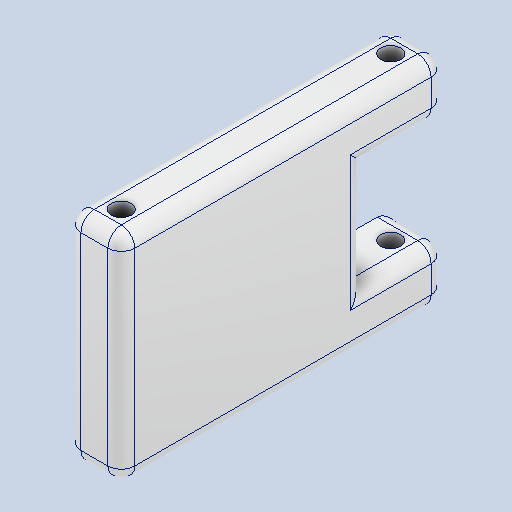
# Autodesk Inventor part: swing pusher
Saved by Autodesk Inventor 2023 (Build 270158000, 158)
## iProperties
Created: 2023-01-25
Part Number: swing pusher
Material: Aluminum 6061
Document SubType Name: Modeling
Designer: Gabriel - T3 CAD
Density: 2.7 g/cm^3
Appearance: Aluminum - Flat
Mass: 108.875 g
Surface Area: 106.324 cm^2
Volume: 40.324 cm^3
Author: Gabriel - T3 CAD
Autodesk Inventor part; units mm, degrees
ref_plane "YZ Plane" through (0, 0, 0) normal (1, 0, 0) x (0, 1, 0)
ref_plane "XZ Plane" through (0, 0, 0) normal (0, 1, 0) x (-1, 0, 0)
ref_plane "XY Plane" through (0, 0, 0) normal (0, 0, 1) x (1, 0, 0)
sketch "Sketch1" plane through (0, 0, 0) normal (0, 1, 0) x (-1, 0, 0)
  line L0 (0, 0) -> (12.7, 0)
  line L1 (12.7, 0) -> (12.7, 76.2)
  line L2 (12.7, 76.2) -> (0, 76.2)
  line L3 (0, 76.2) -> (0, 0)
  circle A0 centre (6.35, 6.35) radius 2.3813
  circle A1 centre (6.35, 69.85) radius 2.3813
  dimension "d0" = 12.7
  dimension "d1" = 76.2
  dimension "d2" = 6.35
  dimension "d3" = 6.35
  dimension "d4" = 4.7625
  dimension "d5" = 6.35
  dimension "d6" = 4.7625
  dimension "d7" = 6.35
  constraints: 8 end point, 2 centre point, 2 parallel, 1 horizontal, 1 perpendicular
  measures "d0" distance of L2.end L1.end
  measures "d1" distance of L1.end L0.end
  measures "d2" distance from line of L0 A0.centre
  measures "d3" distance from line of L1 A0.centre
  measures "d4" diameter of A0
  measures "d5" distance from line of L1 A1.centre
  measures "d6" diameter of A1
  measures "d7" distance from line of L2 A1.centre
extrude "Extrusion1" add sketch "Sketch1" along normal blind 50.8
sketch "Sketch3" plane through (0, 0, 76.2) normal (1, 0, 0) x (0, 0, -1)
  line L0 (76.2, 0) -> (76.2, 50.8) projected
  line L1 (76.2, 38.1) -> (57.15, 38.1)
  line L2 (76.2, 38.1) -> (95.25, 38.1) construction
  line L3 (57.15, 38.1) -> (57.15, 12.7)
  line L4 (57.15, 12.7) -> (76.2, 12.7)
  line L5 (0, 50.8) -> (76.2, 50.8) projected
  line L6 (76.2, 50.8) -> (0, 50.8) projected
  line L7 (57.15, 50.8) -> (57.15, 38.1)
  line L8 (57.15, 12.7) -> (57.15, 0)
  line L9 (76.2, 0) -> (0, 0) projected
  dimension "d24" = 19.05
  dimension "d25" = 180
  dimension "d26" = 25.4
  dimension "d27" = 12.7
  constraints: 12 end point, 5 point on line, 3 perpendicular, 2 collinear, 1 horizontal
  measures "d24" distance of L1.start L1.end
  measures "d25" angle of L1 L2
  measures "d26" distance of L1.end L3.end
  measures "d27" distance between parallel lines of L5 L1
extrude "Extrusion3" cut sketch "Sketch3" against normal through all contours L4 L3 L1 L0
fillet "Fillet1" radius 3.175 21 edges at (0, 50.8, 38.1) (-12.7, 50.8, 38.1) (-6.35, 50.8, 76.2) (0, 0, 38.1) (-12.7, 0, 38.1) (0, 25.4, 76.2) (-12.7, 25.4, 76.2) (-6.35, 0, 76.2) (0, 6.35, 0) (0, 12.7, 9.525) (-6.35, 12.7, 0) (0, 25.4, 19.05) (-12.7, 6.35, 0) (-6.35, 0, 0) (0, 38.1, 9.525) (-6.35, 38.1, 0) (0, 44.45, 0) (-6.35, 50.8, 0) (-12.7, 44.45, 0) (-12.7, 38.1, 9.525) (-12.7, 25.4, 19.05)
body "Solid1"
